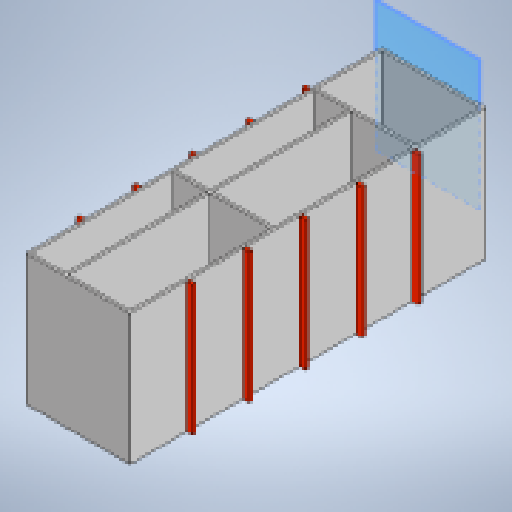
# Autodesk Inventor part: BSH 600 Tank dummy
Saved by Autodesk Inventor 2025.1 (Build 291241020, 241B)
## iProperties
Created: 2024-09-10
Part Number: BSH 600 Tank dummy
Material: Generic
Document SubType Name: Modeling
Designer: admin
Density: 1 g/cm^3
Appearance: Default
Author: admin
Autodesk Inventor part; units mm, degrees
ref_plane "YZ Plane" through (0, 0, 0) normal (1, 0, 0) x (0, 1, 0)
ref_plane "XZ Plane" through (0, 0, 0) normal (0, 1, 0) x (-1, 0, 0)
ref_plane "XY Plane" through (0, 0, 0) normal (0, 0, 1) x (1, 0, 0)
sketch "Sketch1" plane through (0, 0, 0) normal (0, 0, 1) x (1, 0, 0)
  line L0 (1200, 4100) -> (-1200, 4100)
  line L1 (-1200, 4100) -> (-1200, -4100)
  line L2 (-1200, -4100) -> (1200, -4100)
  line L3 (1200, -4100) -> (1200, 4100)
  line L4 (1200, 4100) -> (-1200, -4100) construction
  line L5 (-1200, 4100) -> (1200, -4100) construction
  point P0 (0, 0)
  dimension "d0" = 2400
  dimension "d1" = 8200
  constraints: 12 end point, 2 midpoint, 2 parallel, 1 horizontal, 1 perpendicular
  measures "d0" distance of L2.end L1.end
  measures "d1" distance of L1.end L0.end
extrude "Extrusion1" add sketch "Sketch1" along normal blind 10
sketch "Sketch2" plane through (0, 0, 10) normal (0, 0, 1) x (1, 0, 0)
  line L0 (-1200, 4100) -> (-1200, -4100) projected
  line L1 (-1200, -4100) -> (1200, -4100) projected
  line L2 (1200, -4100) -> (1200, 4100) projected
  line L3 (1200, 4100) -> (-1200, 4100) projected
  line L4 (1140, 4040) -> (1140, -4040)
  line L5 (1140, -4040) -> (-1140, -4040)
  line L6 (-1140, -4040) -> (-1140, 4040)
  line L7 (-1140, 4040) -> (1140, 4040)
  line L8 (1140, 2540) -> (-1140, 2540)
  line L9 (-1140, 2540) -> (-1140, 2480)
  line L10 (-1140, 2480) -> (1140, 2480)
  line L11 (1140, 2480) -> (1140, 2540)
  line L12 (-280, -4040) -> (-340, -4040)
  line L13 (-340, -4040) -> (-340, 2480)
  line L14 (-340, 2480) -> (-280, 2480)
  line L15 (-280, 2480) -> (-280, -4040)
  line L16 (-1140, -720) -> (1140, -720)
  line L17 (1140, -720) -> (1140, -780)
  line L18 (1140, -780) -> (-1140, -780)
  line L19 (-1140, -780) -> (-1140, -720)
  point P0 (0, 0)
  point P1 (-280, -720)
  point P2 (-340, -780)
  point P3 (-1140, -780)
  point P4 (-280, -780)
  point P5 (-340, -720)
  dimension "d4" = 60
  dimension "d5" = 60
  dimension "d6" = 1500
  dimension "d7" = 800
  dimension "d8" = 3200
  constraints: 32 end point, 6 parallel, 5 perpendicular, 4 collinear, 3 horizontal, 2 point on line, 3 other
  measures "d4" distance between parallel lines of L2 L4
  measures "d5" distance between parallel lines of L10 L8
  measures "d6" distance between parallel lines of L8 L7
  measures "d7" distance between parallel lines of L6 L13
  measures "d8" distance between parallel lines of L16 L10
extrude "Extrusion2" add sketch "Sketch2" along normal blind 3000 contours L3 L2 L1 L0 | L4 L10 L6 L8 | L4 L18 L15 L16 | L15 L16 L13 L10 | L15 L18 L13 L16 | L16 L13 L18 L6 | L15 L5 L13 L18
sketch "Sketch3" plane through (0, 0, 0) normal (0, 0, 1) x (1, 0, 0)
  line L0 (-1200, 4100) -> (-1200, -4100) construction
  line L1 (1200, 4100) -> (-1200, 4100) construction
  line L2 (1200, -4100) -> (1200, 4100) construction
  line L3 (-1200, -4100) -> (1200, -4100) construction
  line L4 (-1200, 2480) -> (-1340, 2480)
  line L5 (-1340, 2480) -> (-1340, 2400)
  line L6 (-1340, 2400) -> (-1200, 2400)
  line L7 (-1200, 2400) -> (-1200, 2480)
  line L8 (1200, 2480) -> (1340, 2480)
  line L9 (1340, 2480) -> (1340, 2400)
  line L10 (1340, 2400) -> (1200, 2400)
  line L11 (1200, 2400) -> (1200, 2480)
  point P0 (0, 0)
  dimension "d11" = 140
  dimension "d12" = 80
  dimension "d13" = 1620
  constraints: 16 end point, 4 parallel, 2 equal length, 2 horizontal, 2 perpendicular, 2 point on line, 1 collinear
  measures "d11" distance of L6.end L5.end
  measures "d12" distance of L5.end L4.end
  measures "d13" distance between parallel lines of L1 L4
extrude "Extrusion3" add sketch "Sketch3" along normal blind 3000
pattern_linear "Rectangular Pattern1" count 5 spacing 1300 along (0, -1, 0) of "Extrusion3"
equation "\"d5\" = d4"
body "Solid1"
